Autodesk Fusion 360 part; units mm, degrees
(part 2 of 2)
sketch "Sketch3" plane through (0, 0, 2) normal (0, 0, 1) x (-1, 0, 0)
  line L0 (-59.1799, 22.5268) -> (-59.1799, -21.7585)
  arc A0 (-59.1799, -21.7585) -> (-58.4799, -22.4585) centre (-58.4799, -21.7585) ccw
  line L1 (-58.4799, -22.4585) -> (-40.7999, -22.4585)
  arc A1 (-39.4999, -23.7585) -> (-40.7999, -22.4585) centre (-40.7999, -23.7585) ccw
  line L2 (-39.4999, -23.7585) -> (-39.4999, -31.8337)
  arc A2 (-39.4999, -31.8337) -> (-38.7999, -32.5337) centre (-38.7999, -31.8337) ccw
  line L3 (-38.7999, -32.5337) -> (-21.7399, -32.5337)
  arc A3 (-20.4399, -33.8337) -> (-21.7399, -32.5337) centre (-21.7399, -33.8337) ccw
  line L4 (-20.4399, -33.8337) -> (-20.4399, -41.2137)
  arc A4 (-20.4399, -41.2137) -> (-19.7399, -41.9137) centre (-19.7399, -41.2137) ccw
  line L5 (-19.7399, -41.9137) -> (4.6619, -41.9137)
  arc A5 (4.6619, -41.9137) -> (5.3619, -41.2137) centre (4.6619, -41.2137) ccw
  line L6 (5.3619, -41.2137) -> (5.3619, -33.5689)
  arc A6 (6.6619, -32.2689) -> (5.3619, -33.5689) centre (6.6619, -33.5689) ccw
  line L7 (6.6619, -32.2689) -> (23.7728, -32.2689)
  arc A7 (23.7728, -32.2689) -> (24.4728, -31.5689) centre (23.7728, -31.5689) ccw
  line L8 (24.4728, -31.5689) -> (24.4728, -24.0218)
  arc A8 (25.7728, -22.7218) -> (24.4728, -24.0218) centre (25.7728, -24.0218) ccw
  line L9 (25.7728, -22.7218) -> (43.2453, -22.7218)
  arc A9 (43.2453, -22.7218) -> (43.9453, -22.0218) centre (43.2453, -22.0218) ccw
  line L10 (43.9453, -22.0218) -> (43.9453, -14.2468)
  arc A10 (45.2453, -12.9468) -> (43.9453, -14.2468) centre (45.2453, -14.2468) ccw
  line L11 (45.2453, -12.9468) -> (71.9981, -12.9468)
  arc A11 (71.9981, -12.9468) -> (72.6981, -12.2468) centre (71.9981, -12.2468) ccw
  line L12 (72.6981, -12.2468) -> (72.6981, 55.2276)
  arc A12 (72.6981, 55.2276) -> (71.9981, 55.9276) centre (71.9981, 55.2276) ccw
  line L13 (71.9981, 55.9276) -> (-16.5099, 55.9276)
  arc A13 (-17.8099, 57.2276) -> (-16.5099, 55.9276) centre (-16.5099, 57.2276) ccw
  line L14 (-17.8099, 57.2276) -> (-17.8099, 63.7813)
  arc A14 (-17.8099, 63.7813) -> (-18.5099, 64.4813) centre (-18.5099, 63.7813) ccw
  line L15 (-18.5099, 64.4813) -> (-80.5907, 64.4813)
  arc A15 (-80.5907, 64.4813) -> (-81.2907, 63.7813) centre (-80.5907, 63.7813) ccw
  line L16 (-81.2907, 63.7813) -> (-81.2907, 1.9527)
  arc A16 (-81.2907, 1.9527) -> (-80.5907, 1.2527) centre (-80.5907, 1.9527) ccw
  line L17 (-80.5907, 1.2527) -> (-77.3, 1.2527)
  line L18 (-77.3, 1.2527) -> (-77.3, 22.5268)
  line L19 (-77.3, 22.5268) -> (-59.1799, 22.5268)
  arc A17 (56.3681, 12.1532) -> (56.8681, 12.6532) centre (56.3681, 12.6532) ccw
  line L20 (56.3681, 12.1532) -> (43.3681, 12.1532)
  arc A18 (42.8681, 12.6532) -> (43.3681, 12.1532) centre (43.3681, 12.6532) ccw
  line L21 (42.8681, 12.6532) -> (42.8681, 25.6532)
  arc A19 (43.3681, 26.1532) -> (42.8681, 25.6532) centre (43.3681, 25.6532) ccw
  line L22 (43.3681, 26.1532) -> (56.3681, 26.1532)
  arc A20 (56.8681, 25.6532) -> (56.3681, 26.1532) centre (56.3681, 25.6532) ccw
  line L23 (56.8681, 25.6532) -> (56.8681, 12.6532)
  arc A21 (-0.7819, -16.4218) -> (-0.2819, -15.9218) centre (-0.7819, -15.9218) ccw
  line L24 (-0.7819, -16.4218) -> (-13.7819, -16.4218)
  arc A22 (-14.2819, -15.9218) -> (-13.7819, -16.4218) centre (-13.7819, -15.9218) ccw
  line L25 (-14.2819, -15.9218) -> (-14.2819, -2.9218)
  arc A23 (-13.7819, -2.4218) -> (-14.2819, -2.9218) centre (-13.7819, -2.9218) ccw
  line L26 (-13.7819, -2.4218) -> (-0.7819, -2.4218)
  arc A24 (-0.2819, -2.9218) -> (-0.7819, -2.4218) centre (-0.7819, -2.9218) ccw
  line L27 (-0.2819, -2.9218) -> (-0.2819, -15.9218)
  arc A25 (18.2681, 12.1532) -> (18.7681, 12.6532) centre (18.2681, 12.6532) ccw
  line L28 (18.2681, 12.1532) -> (5.2681, 12.1532)
  arc A26 (4.7681, 12.6532) -> (5.2681, 12.1532) centre (5.2681, 12.6532) ccw
  line L29 (4.7681, 12.6532) -> (4.7681, 25.6532)
  arc A27 (5.2681, 26.1532) -> (4.7681, 25.6532) centre (5.2681, 25.6532) ccw
  line L30 (5.2681, 26.1532) -> (18.2681, 26.1532)
  arc A28 (18.7681, 25.6532) -> (18.2681, 26.1532) centre (18.2681, 25.6532) ccw
  line L31 (18.7681, 25.6532) -> (18.7681, 12.6532)
  arc A29 (56.3681, -6.8968) -> (56.8681, -6.3968) centre (56.3681, -6.3968) ccw
  line L32 (56.3681, -6.8968) -> (43.3681, -6.8968)
  arc A30 (42.8681, -6.3968) -> (43.3681, -6.8968) centre (43.3681, -6.3968) ccw
  line L33 (42.8681, -6.3968) -> (42.8681, 6.6032)
  arc A31 (43.3681, 7.1032) -> (42.8681, 6.6032) centre (43.3681, 6.6032) ccw
  line L34 (43.3681, 7.1032) -> (56.3681, 7.1032)
  arc A32 (56.8681, 6.6032) -> (56.3681, 7.1032) centre (56.3681, 6.6032) ccw
  line L35 (56.8681, 6.6032) -> (56.8681, -6.3968)
  arc A33 (18.2681, -6.8968) -> (18.7681, -6.3968) centre (18.2681, -6.3968) ccw
  line L36 (18.2681, -6.8968) -> (5.2681, -6.8968)
  arc A34 (4.7681, -6.3968) -> (5.2681, -6.8968) centre (5.2681, -6.3968) ccw
  line L37 (4.7681, -6.3968) -> (4.7681, 6.6032)
  arc A35 (5.2681, 7.1032) -> (4.7681, 6.6032) centre (5.2681, 6.6032) ccw
  line L38 (5.2681, 7.1032) -> (18.2681, 7.1032)
  arc A36 (18.7681, 6.6032) -> (18.2681, 7.1032) centre (18.2681, 6.6032) ccw
  line L39 (18.7681, 6.6032) -> (18.7681, -6.3968)
  arc A37 (-38.8819, 2.6282) -> (-38.3819, 3.1282) centre (-38.8819, 3.1282) ccw
  line L40 (-38.8819, 2.6282) -> (-51.8819, 2.6282)
  arc A38 (-52.3819, 3.1282) -> (-51.8819, 2.6282) centre (-51.8819, 3.1282) ccw
  line L41 (-52.3819, 3.1282) -> (-52.3819, 16.1282)
  arc A39 (-51.8819, 16.6282) -> (-52.3819, 16.1282) centre (-51.8819, 16.1282) ccw
  line L42 (-51.8819, 16.6282) -> (-38.8819, 16.6282)
  arc A40 (-38.3819, 16.1282) -> (-38.8819, 16.6282) centre (-38.8819, 16.1282) ccw
  line L43 (-38.3819, 16.1282) -> (-38.3819, 3.1282)
  arc A41 (-19.8319, 31.2032) -> (-19.3319, 31.7032) centre (-19.8319, 31.7032) ccw
  line L44 (-19.8319, 31.2032) -> (-32.8319, 31.2032)
  arc A42 (-33.3319, 31.7032) -> (-32.8319, 31.2032) centre (-32.8319, 31.7032) ccw
  line L45 (-33.3319, 31.7032) -> (-33.3319, 44.7032)
  arc A43 (-32.8319, 45.2032) -> (-33.3319, 44.7032) centre (-32.8319, 44.7032) ccw
  line L46 (-32.8319, 45.2032) -> (-19.8319, 45.2032)
  arc A44 (-19.3319, 44.7032) -> (-19.8319, 45.2032) centre (-19.8319, 44.7032) ccw
  line L47 (-19.3319, 44.7032) -> (-19.3319, 31.7032)
  arc A45 (37.3181, 2.6282) -> (37.8181, 3.1282) centre (37.3181, 3.1282) ccw
  line L48 (37.3181, 2.6282) -> (24.3181, 2.6282)
  arc A46 (23.8181, 3.1282) -> (24.3181, 2.6282) centre (24.3181, 3.1282) ccw
  line L49 (23.8181, 3.1282) -> (23.8181, 16.1282)
  arc A47 (24.3181, 16.6282) -> (23.8181, 16.1282) centre (24.3181, 16.1282) ccw
  line L50 (24.3181, 16.6282) -> (37.3181, 16.6282)
  arc A48 (37.8181, 16.1282) -> (37.3181, 16.6282) centre (37.3181, 16.1282) ccw
  line L51 (37.8181, 16.1282) -> (37.8181, 3.1282)
  arc A49 (-38.8819, 40.7282) -> (-38.3819, 41.2282) centre (-38.8819, 41.2282) ccw
  line L52 (-38.8819, 40.7282) -> (-51.8819, 40.7282)
  arc A50 (-52.3819, 41.2282) -> (-51.8819, 40.7282) centre (-51.8819, 41.2282) ccw
  line L53 (-52.3819, 41.2282) -> (-52.3819, 54.2282)
  arc A51 (-51.8819, 54.7282) -> (-52.3819, 54.2282) centre (-51.8819, 54.2282) ccw
  line L54 (-51.8819, 54.7282) -> (-38.8819, 54.7282)
  arc A52 (-38.3819, 54.2282) -> (-38.8819, 54.7282) centre (-38.8819, 54.2282) ccw
  line L55 (-38.3819, 54.2282) -> (-38.3819, 41.2282)
  arc A53 (-38.8819, -16.4218) -> (-38.3819, -15.9218) centre (-38.8819, -15.9218) ccw
  line L56 (-38.8819, -16.4218) -> (-51.8819, -16.4218)
  arc A54 (-52.3819, -15.9218) -> (-51.8819, -16.4218) centre (-51.8819, -15.9218) ccw
  line L57 (-52.3819, -15.9218) -> (-52.3819, -2.9218)
  arc A55 (-51.8819, -2.4218) -> (-52.3819, -2.9218) centre (-51.8819, -2.9218) ccw
  line L58 (-51.8819, -2.4218) -> (-38.8819, -2.4218)
  arc A56 (-38.3819, -2.9218) -> (-38.8819, -2.4218) centre (-38.8819, -2.9218) ccw
  line L59 (-38.3819, -2.9218) -> (-38.3819, -15.9218)
  arc A57 (-19.8319, -25.9468) -> (-19.3319, -25.4468) centre (-19.8319, -25.4468) ccw
  line L60 (-19.8319, -25.9468) -> (-32.8319, -25.9468)
  arc A58 (-33.3319, -25.4468) -> (-32.8319, -25.9468) centre (-32.8319, -25.4468) ccw
  line L61 (-33.3319, -25.4468) -> (-33.3319, -12.4468)
  arc A59 (-32.8319, -11.9468) -> (-33.3319, -12.4468) centre (-32.8319, -12.4468) ccw
  line L62 (-32.8319, -11.9468) -> (-19.8319, -11.9468)
  arc A60 (-19.3319, -12.4468) -> (-19.8319, -11.9468) centre (-19.8319, -12.4468) ccw
  line L63 (-19.3319, -12.4468) -> (-19.3319, -25.4468)
  arc A61 (-19.8319, 12.1532) -> (-19.3319, 12.6532) centre (-19.8319, 12.6532) ccw
  line L64 (-19.8319, 12.1532) -> (-32.8319, 12.1532)
  arc A62 (-33.3319, 12.6532) -> (-32.8319, 12.1532) centre (-32.8319, 12.6532) ccw
  line L65 (-33.3319, 12.6532) -> (-33.3319, 25.6532)
  arc A63 (-32.8319, 26.1532) -> (-33.3319, 25.6532) centre (-32.8319, 25.6532) ccw
  line L66 (-32.8319, 26.1532) -> (-19.8319, 26.1532)
  arc A64 (-19.3319, 25.6532) -> (-19.8319, 26.1532) centre (-19.8319, 25.6532) ccw
  line L67 (-19.3319, 25.6532) -> (-19.3319, 12.6532)
  arc A65 (37.3181, -16.4218) -> (37.8181, -15.9218) centre (37.3181, -15.9218) ccw
  line L68 (37.3181, -16.4218) -> (24.3181, -16.4218)
  arc A66 (23.8181, -15.9218) -> (24.3181, -16.4218) centre (24.3181, -15.9218) ccw
  line L69 (23.8181, -15.9218) -> (23.8181, -2.9218)
  arc A67 (24.3181, -2.4218) -> (23.8181, -2.9218) centre (24.3181, -2.9218) ccw
  line L70 (24.3181, -2.4218) -> (37.3181, -2.4218)
  arc A68 (37.8181, -2.9218) -> (37.3181, -2.4218) centre (37.3181, -2.9218) ccw
  line L71 (37.8181, -2.9218) -> (37.8181, -15.9218)
  arc A69 (56.3681, 31.2032) -> (56.8681, 31.7032) centre (56.3681, 31.7032) ccw
  line L72 (56.3681, 31.2032) -> (43.3681, 31.2032)
  arc A70 (42.8681, 31.7032) -> (43.3681, 31.2032) centre (43.3681, 31.7032) ccw
  line L73 (42.8681, 31.7032) -> (42.8681, 44.7032)
  arc A71 (43.3681, 45.2032) -> (42.8681, 44.7032) centre (43.3681, 44.7032) ccw
  line L74 (43.3681, 45.2032) -> (56.3681, 45.2032)
  arc A72 (56.8681, 44.7032) -> (56.3681, 45.2032) centre (56.3681, 44.7032) ccw
  line L75 (56.8681, 44.7032) -> (56.8681, 31.7032)
  arc A73 (-19.8319, -6.8968) -> (-19.3319, -6.3968) centre (-19.8319, -6.3968) ccw
  line L76 (-19.8319, -6.8968) -> (-32.8319, -6.8968)
  arc A74 (-33.3319, -6.3968) -> (-32.8319, -6.8968) centre (-32.8319, -6.3968) ccw
  line L77 (-33.3319, -6.3968) -> (-33.3319, 6.6032)
  arc A75 (-32.8319, 7.1032) -> (-33.3319, 6.6032) centre (-32.8319, 6.6032) ccw
  line L78 (-32.8319, 7.1032) -> (-19.8319, 7.1032)
  arc A76 (-19.3319, 6.6032) -> (-19.8319, 7.1032) centre (-19.8319, 6.6032) ccw
  line L79 (-19.3319, 6.6032) -> (-19.3319, -6.3968)
  arc A77 (-0.7819, 2.6282) -> (-0.2819, 3.1282) centre (-0.7819, 3.1282) ccw
  line L80 (-0.7819, 2.6282) -> (-13.7819, 2.6282)
  arc A78 (-14.2819, 3.1282) -> (-13.7819, 2.6282) centre (-13.7819, 3.1282) ccw
  line L81 (-14.2819, 3.1282) -> (-14.2819, 16.1282)
  arc A79 (-13.7819, 16.6282) -> (-14.2819, 16.1282) centre (-13.7819, 16.1282) ccw
  line L82 (-13.7819, 16.6282) -> (-0.7819, 16.6282)
  arc A80 (-0.2819, 16.1282) -> (-0.7819, 16.6282) centre (-0.7819, 16.1282) ccw
  line L83 (-0.2819, 16.1282) -> (-0.2819, 3.1282)
  arc A81 (18.2681, -25.9468) -> (18.7681, -25.4468) centre (18.2681, -25.4468) ccw
  line L84 (18.2681, -25.9468) -> (5.2681, -25.9468)
  arc A82 (4.7681, -25.4468) -> (5.2681, -25.9468) centre (5.2681, -25.4468) ccw
  line L85 (4.7681, -25.4468) -> (4.7681, -12.4468)
  arc A83 (5.2681, -11.9468) -> (4.7681, -12.4468) centre (5.2681, -12.4468) ccw
  line L86 (5.2681, -11.9468) -> (18.2681, -11.9468)
  arc A84 (18.7681, -12.4468) -> (18.2681, -11.9468) centre (18.2681, -12.4468) ccw
  line L87 (18.7681, -12.4468) -> (18.7681, -25.4468)
  arc A85 (-0.7819, 21.6782) -> (-0.2819, 22.1782) centre (-0.7819, 22.1782) ccw
  line L88 (-0.7819, 21.6782) -> (-13.7819, 21.6782)
  arc A86 (-14.2819, 22.1782) -> (-13.7819, 21.6782) centre (-13.7819, 22.1782) ccw
  line L89 (-14.2819, 22.1782) -> (-14.2819, 35.1782)
  arc A87 (-13.7819, 35.6782) -> (-14.2819, 35.1782) centre (-13.7819, 35.1782) ccw
  line L90 (-13.7819, 35.6782) -> (-0.7819, 35.6782)
  arc A88 (-0.2819, 35.1782) -> (-0.7819, 35.6782) centre (-0.7819, 35.1782) ccw
  line L91 (-0.2819, 35.1782) -> (-0.2819, 22.1782)
  arc A89 (-0.7819, -35.4718) -> (-0.2819, -34.9718) centre (-0.7819, -34.9718) ccw
  line L92 (-0.7819, -35.4718) -> (-13.7819, -35.4718)
  arc A90 (-14.2819, -34.9718) -> (-13.7819, -35.4718) centre (-13.7819, -34.9718) ccw
  line L93 (-14.2819, -34.9718) -> (-14.2819, -21.9718)
  arc A91 (-13.7819, -21.4718) -> (-14.2819, -21.9718) centre (-13.7819, -21.9718) ccw
  line L94 (-13.7819, -21.4718) -> (-0.7819, -21.4718)
  arc A92 (-0.2819, -21.9718) -> (-0.7819, -21.4718) centre (-0.7819, -21.9718) ccw
  line L95 (-0.2819, -21.9718) -> (-0.2819, -34.9718)
  arc A93 (37.3181, 21.6782) -> (37.8181, 22.1782) centre (37.3181, 22.1782) ccw
  line L96 (37.3181, 21.6782) -> (24.3181, 21.6782)
  arc A94 (23.8181, 22.1782) -> (24.3181, 21.6782) centre (24.3181, 22.1782) ccw
  line L97 (23.8181, 22.1782) -> (23.8181, 35.1782)
  arc A95 (24.3181, 35.6782) -> (23.8181, 35.1782) centre (24.3181, 35.1782) ccw
  line L98 (24.3181, 35.6782) -> (37.3181, 35.6782)
  arc A96 (37.8181, 35.1782) -> (37.3181, 35.6782) centre (37.3181, 35.1782) ccw
  line L99 (37.8181, 35.1782) -> (37.8181, 22.1782)
  arc A97 (-38.8819, 21.6782) -> (-38.3819, 22.1782) centre (-38.8819, 22.1782) ccw
  line L100 (-38.8819, 21.6782) -> (-51.8819, 21.6782)
  arc A98 (-52.3819, 22.1782) -> (-51.8819, 21.6782) centre (-51.8819, 22.1782) ccw
  line L101 (-52.3819, 22.1782) -> (-52.3819, 35.1782)
  arc A99 (-51.8819, 35.6782) -> (-52.3819, 35.1782) centre (-51.8819, 35.1782) ccw
  line L102 (-51.8819, 35.6782) -> (-38.8819, 35.6782)
  arc A100 (-38.3819, 35.1782) -> (-38.8819, 35.6782) centre (-38.8819, 35.1782) ccw
  line L103 (-38.3819, 35.1782) -> (-38.3819, 22.1782)
  line L104 (-72.4807, 57.9) -> (-69.7, 57.9)
  line L105 (-69.7, 57.9) -> (-69.7, 53.3)
  line L106 (-69.7, 53.3) -> (-74.2, 53.3)
  line L107 (-74.2, 53.3) -> (-74.2, 56.0978)
  line L108 (-74.2, 56.0978) -> (-75.5, 56.0978)
  line L109 (-75.5, 56.0978) -> (-75.5, 53)
  spline S0 degree 5 poles (-75.5, 53) (-75.502, 52.9979) (-75.5051, 52.9917) (-75.5078, 52.9763) (-75.5069, 52.9435) (-75.4984, 52.8833) (-75.4821, 52.8077) (-75.457, 52.7235) (-75.4225, 52.6381) (-75.3783, 52.5575) (-75.3249, 52.4843) (-75.2638, 52.417) (-75.1966, 52.3524) (-75.1249, 52.2868) (-75.0495, 52.2181) (-74.9704, 52.1461) (-74.887, 52.0719) (-74.7988, 51.9974) (-74.7051, 51.925) (-74.6059, 51.8566) (-74.5013, 51.7939) (-74.3919, 51.7381) (-74.2782, 51.6893) (-74.1608, 51.6467) (-74.0404, 51.6082) (-73.9181, 51.5712) (-73.7955, 51.5333) (-73.6751, 51.4924) (-73.5605, 51.448) (-73.4569, 51.4009) (-73.3693, 51.353) (-73.3019, 51.3058) (-73.2568, 51.2606) (-73.2332, 51.2167) (-73.2281, 51.1723) (-73.2385, 51.1244) (-73.2623, 51.069) (-73.2986, 51.0022) (-73.3469, 50.9211) (-73.4063, 50.8255) (-73.476, 50.7172) (-73.5547, 50.5999) (-73.6412, 50.4774) (-73.734, 50.3537) (-73.8318, 50.2312) (-73.9336, 50.1108) (-74.0379, 49.9924) (-74.1434, 49.8754) (-74.2483, 49.7592) (-74.3503, 49.6435) (-74.4466, 49.529) (-74.534, 49.4175) (-74.6095, 49.311) (-74.6709, 49.2111) (-74.7174, 49.1183) (-74.7503, 49.0314) (-74.773, 48.9474) (-74.7898, 48.8621) (-74.8049, 48.7712) (-74.8214, 48.6709) (-74.8405, 48.5587) (-74.8621, 48.4329) (-74.8856, 48.2927) (-74.91, 48.1379) (-74.9348, 47.9691) (-74.9599, 47.7873) (-74.9857, 47.5941) (-75.0127, 47.391) (-75.0417, 47.1799) (-75.0736, 46.9629) (-75.1088, 46.7416) (-75.1478, 46.5178) (-75.1906, 46.2926) (-75.2371, 46.0673) (-75.2868, 45.8426) (-75.3393, 45.6193) (-75.3942, 45.3977) (-75.4512, 45.1783) (-75.5101, 44.9612) (-75.5708, 44.7465) (-75.634, 44.5344) (-75.6999, 44.3248) (-75.7694, 44.1179) (-75.8431, 43.9138) (-75.9213, 43.713) (-76.0045, 43.5159) (-76.0924, 43.3234) (-76.1845, 43.1368) (-76.2799, 42.9574) (-76.377, 42.7869) (-76.4745, 42.6271) (-76.5706, 42.4797) (-76.664, 42.3464) (-76.7533, 42.2283) (-76.8375, 42.1264) (-76.9163, 42.0413) (-76.9746, 41.9868) (-77.0158, 41.9536) (-77.042, 41.9348) (-77.0548, 41.9263) knots -1 -1 -1 -1 -1 -1 -0.98947368 -0.97894737 -0.96842105 -0.95789474 -0.94736842 -0.93684211 -0.92631579 -0.91578947 -0.90526316 -0.89473684 -0.88421053 -0.87368421 -0.86315789 -0.85263158 -0.84210526 -0.83157895 -0.82105263 -0.81052632 -0.8 -0.78947368 -0.77894737 -0.76842105 -0.75789474 -0.74736842 -0.73684211 -0.72631579 -0.71578947 -0.70526316 -0.69473684 -0.68421053 -0.67368421 -0.66315789 -0.65263158 -0.64210526 -0.63157895 -0.62105263 -0.61052632 -0.6 -0.58947368 -0.57894737 -0.56842105 -0.55789474 -0.54736842 -0.53684211 -0.52631579 -0.51578947 -0.50526316 -0.49473684 -0.48421053 -0.47368421 -0.46315789 -0.45263158 -0.44210526 -0.43157895 -0.42105263 -0.41052632 -0.4 -0.38947368 -0.37894737 -0.36842105 -0.35789474 -0.34736842 -0.33684211 -0.32631579 -0.31578947 -0.30526316 -0.29473684 -0.28421053 -0.27368421 -0.26315789 -0.25263158 -0.24210526 -0.23157895 -0.22105263 -0.21052632 -0.2 -0.18947368 -0.17894737 -0.16842105 -0.15789474 -0.14736842 -0.13684211 -0.12631579 -0.11578947 -0.10526316 -0.09473684 -0.08421053 -0.07368421 -0.06315789 -0.05263158 -0.04210526 -0.03157895 -0.02105263 -0.01052632 0 0 0 0 0 0
  line L110 (-77.0548, 41.9263) -> (-77.0548, 56.0876)
  line L111 (-77.0548, 56.0876) -> (-78.5, 56.0876)
  line L112 (-78.5, 56.0876) -> (-78.5, 40.3)
  line L113 (-78.5, 40.3) -> (-79.9, 40.3)
  line L114 (-79.9, 40.3) -> (-79.9, 57.9)
  line L115 (-79.9, 57.9) -> (-77.05, 57.9)
  line L116 (-77.05, 57.9) -> (-77.05, 59.25)
  line L117 (-77.05, 59.25) -> (-79.9, 59.25)
  line L118 (-79.9, 59.25) -> (-79.9, 63.65)
  line L119 (-79.9, 63.65) -> (-75.5, 63.65)
  line L120 (-75.5, 63.65) -> (-75.5, 60.7)
  line L121 (-75.5, 60.7) -> (-74.2, 60.7)
  line L122 (-74.2, 60.7) -> (-74.2, 63.65)
  line L123 (-74.2, 63.65) -> (-56.6, 63.65)
  line L124 (-56.6, 63.65) -> (-56.6, 62)
  line L125 (-56.6, 62) -> (-72.4, 62)
  line L126 (-72.4, 62) -> (-72.4, 60.7)
  line L127 (-72.4, 60.7) -> (-58.5, 60.7)
  spline S1 degree 5 poles (-58.5, 60.7) (-58.4979, 60.6989) (-58.4916, 60.6972) (-58.4761, 60.696) (-58.4433, 60.6972) (-58.3845, 60.7015) (-58.3157, 60.7034) (-58.2511, 60.694) (-58.2036, 60.667) (-58.1802, 60.6236) (-58.176, 60.5775) (-58.1828, 60.5435) (-58.1973, 60.5256) (-58.2263, 60.5108) (-58.2788, 60.4818) (-58.3601, 60.4282) (-58.47, 60.3489) (-58.6052, 60.2482) (-58.7602, 60.1344) (-58.9288, 60.0167) (-59.1052, 59.9038) (-59.2855, 59.8005) (-59.4676, 59.7089) (-59.6507, 59.6284) (-59.8349, 59.557) (-60.0207, 59.4919) (-60.209, 59.4296) (-60.4006, 59.3672) (-60.5954, 59.303) (-60.7931, 59.2365) (-60.9926, 59.168) (-61.1928, 59.0988) (-61.3926, 59.0303) (-61.591, 58.9644) (-61.7875, 58.9026) (-61.9822, 58.846) (-62.176, 58.7953) (-62.3702, 58.7503) (-62.5667, 58.7106) (-62.7668, 58.6755) (-62.9719, 58.6439) (-63.1824, 58.6148) (-63.3979, 58.5873) (-63.6167, 58.5607) (-63.8356, 58.5344) (-64.0509, 58.5082) (-64.2586, 58.4818) (-64.4553, 58.455) (-64.6383, 58.4278) (-64.8063, 58.3998) (-64.96, 58.3706) (-65.1027, 58.3397) (-65.2389, 58.3062) (-65.3733, 58.2695) (-65.51, 58.229) (-65.6509, 58.1843) (-65.7948, 58.1354) (-65.9371, 58.0827) (-66.0718, 58.0267) (-66.1928, 57.9679) (-66.2958, 57.9066) (-66.3798, 57.8428) (-66.4488, 57.776) (-66.5101, 57.7055) (-66.5721, 57.6306) (-66.6423, 57.5514) (-66.7251, 57.469) (-66.8214, 57.3855) (-66.9295, 57.3039) (-67.0459, 57.228) (-67.1662, 57.1621) (-67.2855, 57.1112) (-67.3994, 57.0802) (-67.5043, 57.0731) (-67.5978, 57.0918) (-67.6795, 57.1359) (-67.7513, 57.2008) (-67.8166, 57.2803) (-67.8788, 57.3681) (-67.9408, 57.4597) (-68.0035, 57.5546) (-68.0658, 57.6559) (-68.126, 57.7676) (-68.1819, 57.8935) (-68.2323, 58.0348) (-68.2775, 58.1878) (-68.3192, 58.3449) (-68.36, 58.4969) (-68.4028, 58.6344) (-68.4499, 58.75) (-68.5032, 58.8401) (-68.5627, 58.9072) (-68.6276, 58.9575) (-68.6965, 58.9988) (-68.7682, 59.0385) (-68.8418, 59.0809) (-68.9018, 59.1187) (-68.9475, 59.1496) (-68.9782, 59.1714) (-68.9937, 59.1825) knots -1 -1 -1 -1 -1 -1 -0.98947368 -0.97894737 -0.96842105 -0.95789474 -0.94736842 -0.93684211 -0.92631579 -0.91578947 -0.90526316 -0.89473684 -0.88421053 -0.87368421 -0.86315789 -0.85263158 -0.84210526 -0.83157895 -0.82105263 -0.81052632 -0.8 -0.78947368 -0.77894737 -0.76842105 -0.75789474 -0.74736842 -0.73684211 -0.72631579 -0.71578947 -0.70526316 -0.69473684 -0.68421053 -0.67368421 -0.66315789 -0.65263158 -0.64210526 -0.63157895 -0.62105263 -0.61052632 -0.6 -0.58947368 -0.57894737 -0.56842105 -0.55789474 -0.54736842 -0.53684211 -0.52631579 -0.51578947 -0.50526316 -0.49473684 -0.48421053 -0.47368421 -0.46315789 -0.45263158 -0.44210526 -0.43157895 -0.42105263 -0.41052632 -0.4 -0.38947368 -0.37894737 -0.36842105 -0.35789474 -0.34736842 -0.33684211 -0.32631579 -0.31578947 -0.30526316 -0.29473684 -0.28421053 -0.27368421 -0.26315789 -0.25263158 -0.24210526 -0.23157895 -0.22105263 -0.21052632 -0.2 -0.18947368 -0.17894737 -0.16842105 -0.15789474 -0.14736842 -0.13684211 -0.12631579 -0.11578947 -0.10526316 -0.09473684 -0.08421053 -0.07368421 -0.06315789 -0.05263158 -0.04210526 -0.03157895 -0.02105263 -0.01052632 0 0 0 0 0 0
  line L128 (-68.9937, 59.1825) -> (-72.4807, 59.1825)
  line L129 (-72.4807, 59.1825) -> (-72.4807, 57.9)
  line L130 (43.8051, 55.9276) -> (-3.8051, 55.9276) construction
  line L131 (-3.8051, 55.9276) -> (-3.8051, 44.0724) construction
  line L132 (-3.8051, 44.0724) -> (43.8051, 44.0724) construction
  line L133 (43.8051, 44.0724) -> (43.8051, 55.9276) construction
  dimension "d31" = 3.5
  dimension "d32" = 0
  text T0 "Made with <3 by Anay" font "Impact" height 3.5 align centre middle in box 47.6101 x 11.8551 at (43.8051, 55.9276) x (-1, 0) y (0, -1) spacing 1
  constraint coincident L13
extrude "Extrude3" add sketch "Sketch3" along normal blind 0.5 text T0
equation "d32 = 'Made with <3 by Anay'"
